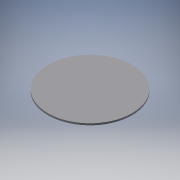
# Autodesk Inventor part: part101
Saved by Autodesk Inventor 2016 (Build 200138000, 138)
## iProperties
Created: 2016-09-06
Part Number: part101
Material: Aluminum 6061
Document SubType Name: Modeling
Designer: gus
Density: 2.7 g/cm^3
Appearance: Aluminum - Flat
Author: gus
Autodesk Inventor part; units mm, degrees
ref_plane "YZ Plane" through (0, 0, 0) normal (1, 0, 0) x (0, 1, 0)
ref_plane "XZ Plane" through (0, 0, 0) normal (0, 1, 0) x (-1, 0, 0)
ref_plane "XY Plane" through (0, 0, 0) normal (0, 0, 1) x (1, 0, 0)
sketch "Sketch1" plane through (0, 0, 0) normal (0, 1, 0) x (-1, 0, 0)
  circle A0 centre (0, 0) radius 152.4
  dimension "d0" = 304.8
  constraints: 1 centre point, 1 coincident
  measures "d0" diameter of A0
extrude "Extrusion1" add sketch "Sketch1" along normal blind 6.35
body "Solid1"
